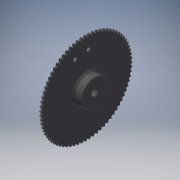
# Autodesk Inventor part: NK35B75_()
Saved by Autodesk Inventor 2018 (Build 220112000, 112)
## iProperties
Category: PARTsolutions
Company: KANA
Created: 2017-10-03
Part Number: NK35B75_()
Catalog Web Link: www.cadenas.de
Description: NK35B-Un-finished
Vendor: KANA
Document SubType Name: Modeling
Designer: psAdmin
Manufacturer: KANA
Mass: 244.907 g
Surface Area: 898.004 cm^2
Volume: 244.907 cm^3
Density: 1 g/cm^3
Material: 一般
Appearance: PSOLRGB-175-175-175
PSOL_IDENT_0: {$CADENAS_DATA\23d-libs\kana\sprockets\chain_no_35\un_finished_sprocket_steel\b_type\nk35b.prj},164
PSOL_IDENT_1: {VTYP=3D},{NB=NK35B75_()},{LINA=NK35B75},{NN=NK35B},{DATE=04.08.2017 01:43:57},{GEOMDATE=30.03.2017
PSOL_IDENT_2: 11:05:00},{VERSION=},{LINEID=490},{LINESUBID=-1},{WBVAR=SURFT}  {NB=NK35B75_()},{LINA=NK35B75},{KT=D
PSOL_IDENT_3: UMMY},{ORDERNO=NK35B75},{TYPE=NK35B},{NOT=75},{NOTX=75.000},{DP=227.46},{DO=233},{DC=222.38},{DC2=22
PSOL_IDENT_4: 2.33},{T=4.3},{DR=5.08},{MAT=None},{MATC=},{SHAPE=W : Welding type},{SHAPENB=W},{SD=16},{SURFT=},{SU
PSOL_IDENT_5: RFTNB=},{BD=68.0},{BL=25},{GD=0},{GDX=0},{S=0},{X=4},{VS=2},{SVDEL1=12},{SVDEL4=42},{SVDEL5=5},{DCX2=
PSOL_IDENT_6: 1}
NN: NK35B
NT: Un-finished
NB: NK35B75_()
NBSYN: NK35B$NOT._($SURFT.)
LINA: NK35B75
TYPE: NK35B
NOT: 75
DP: 227.46
DO: 233
DC: 222.38
DC2: 222.33
T: 4.3
SHAPE: W : Welding type
SD: 16
SURFT: No symbol : No
SUPPLIER: KANA
ARTICLENO: NK35B75_()
BOMINFO: NK35B75
CREATOR: CADENAS GmbH
Title: NK35B75
Author: Cadenas PARTsolutions
Comments: Un-finished
Autodesk Inventor part; units mm, degrees
ref_plane "YZ Plane" through (0, 0, 0) normal (1, 0, 0) x (0, 1, 0)
ref_plane "XZ Plane" through (0, 0, 0) normal (0, 1, 0) x (-1, 0, 0)
ref_plane "XY Plane" through (0, 0, 0) normal (0, 0, 1) x (1, 0, 0)
sketch "Sketch_5" plane through (0, 0, 0) normal (0, 0, 1) x (1, 0, 0)
  line L0 (25, 0) -> (0, 0)
  line L1 (0, 8.9617) -> (0.9617, 8)
  line L2 (0.9617, 8) -> (24.0383, 8)
  line L3 (24.0383, 8) -> (25, 8.9617)
  line L4 (25, 8.9617) -> (25, 33.0383)
  line L5 (25, 33.0383) -> (24.0383, 34)
  line L6 (24.0383, 34) -> (8.3, 34)
  line L7 (8.3, 34) -> (4.3, 38)
  line L8 (4.3, 38) -> (4.3, 114.8906)
  arc A0 (4.3, 114.8906) -> (3.225, 116.5) centre (-0.3844, 112.9253) ccw
  line L9 (3.225, 116.5) -> (1.075, 116.5)
  arc A1 (1.075, 116.5) -> (0, 114.8906) centre (4.6844, 112.9253) ccw
  line L10 (0, 114.8906) -> (0, 8.9617)
  constraints: 22 end point, 4 point on circle, 2 centre point
revolve "Revolution1" add sketch "Sketch_5" angle 360 about axis through (25, 0, 0) along (1, 0, 0)
sketch "Sketch_7" plane through (2.15, 0, 0) normal (1, 0, 0) x (0, 0, -1)
  circle A0 centre (0, 0) radius 155.3333
  arc A1 (-116.4803, -2.1398) -> (-116.4678, -2.7397) centre (0, 0) ccw
  line L0 (-116.4678, -2.7397) -> (-112.3345, -4.8872)
  arc A2 (-112.0613, -9.2305) -> (-112.3345, -4.8872) centre (-113.5056, -7.1412) ccw
  line L1 (-112.0613, -9.2305) -> (-115.8928, -11.8792)
  arc A3 (-115.8928, -11.8792) -> (-115.8301, -12.4759) centre (0, 0) ccw
  line L2 (-115.8301, -12.4759) -> (-111.5316, -14.27)
  arc A4 (-110.8958, -18.5752) -> (-111.5316, -14.27) centre (-112.5099, -16.614) ccw
  line L3 (-110.8958, -18.5752) -> (-114.4923, -21.5352)
  arc A5 (-114.4923, -21.5352) -> (-114.3799, -22.1245) centre (0, 0) ccw
  line L4 (-114.3799, -22.1245) -> (-109.9463, -23.5527)
  arc A6 (-108.9526, -27.7896) -> (-109.9463, -23.5527) centre (-110.7251, -25.9703) ccw
  line L5 (-108.9526, -27.7896) -> (-112.2887, -31.0401)
  arc A7 (-112.2887, -31.0401) -> (-112.1274, -31.618) centre (0, 0) ccw
  line L6 (-112.1274, -31.618) -> (-107.5899, -32.6702)
  arc A8 (-106.2451, -36.8091) -> (-107.5899, -32.6702) centre (-108.1637, -35.1445) ccw
  line L7 (-106.2451, -36.8091) -> (-109.2976, -40.3273)
  arc A9 (-109.2976, -40.3273) -> (-109.0884, -40.8897) centre (0, 0) ccw
  line L8 (-109.0884, -40.8897) -> (-104.4788, -41.5585)
  arc A10 (-102.7924, -45.5703) -> (-104.4788, -41.5585) centre (-104.8435, -44.0721) ccw
  line L9 (-102.7924, -45.5703) -> (-105.5397, -49.3317)
  arc A11 (-105.5397, -49.3317) -> (-105.2843, -49.8746) centre (0, 0) ccw
  line L10 (-105.2843, -49.8746) -> (-100.6349, -50.1553)
  arc A12 (-98.6186, -54.0119) -> (-100.6349, -50.1553) centre (-100.7879, -52.6907) ccw
  line L11 (-98.6186, -54.0119) -> (-101.0416, -57.99)
  arc A13 (-101.0416, -57.99) -> (-100.7416, -58.5096) centre (0, 0) ccw
  line L12 (-100.7416, -58.5096) -> (-96.085, -58.4003)
  arc A14 (-93.7532, -62.0747) -> (-96.085, -58.4003) centre (-96.0254, -60.9396) ccw
  line L13 (-93.7532, -62.0747) -> (-95.8348, -66.2416)
  arc A15 (-95.8348, -66.2416) -> (-95.4924, -66.7343) centre (0, 0) ccw
  line L14 (-95.4924, -66.7343) -> (-90.8612, -66.2357)
  arc A16 (-88.2301, -69.7021) -> (-90.8612, -66.2357) centre (-90.5893, -68.7611) ccw
  line L15 (-88.2301, -69.7021) -> (-89.9557, -74.0285)
  arc A17 (-89.9557, -74.0285) -> (-89.5733, -74.4908) centre (0, 0) ccw
  line L16 (-89.5733, -74.4908) -> (-85.0001, -73.6064)
  arc A18 (-82.0881, -76.8405) -> (-85.0001, -73.6064) centre (-84.5179, -76.1002) ccw
  line L17 (-82.0881, -76.8405) -> (-83.4457, -81.2962)
  arc A19 (-83.4457, -81.2962) -> (-83.0259, -81.7249) centre (0, 0) ccw
  line L18 (-83.0259, -81.7249) -> (-78.5428, -80.4609)
  arc A20 (-75.3704, -83.44) -> (-78.5428, -80.4609) centre (-77.8535, -82.9056) ccw
  line L19 (-75.3704, -83.44) -> (-76.3503, -87.9936)
  arc A21 (-76.3503, -87.9936) -> (-75.8961, -88.3857) centre (0, 0) ccw
  line L20 (-75.8961, -88.3857) -> (-71.5345, -86.751)
  arc A22 (-68.124, -89.4542) -> (-71.5345, -86.751) centre (-70.6431, -89.1295) ccw
  line L21 (-68.124, -89.4542) -> (-68.7195, -94.0738)
  arc A23 (-68.7195, -94.0738) -> (-68.234, -94.4265) centre (0, 0) ccw
  line L22 (-68.234, -94.4265) -> (-64.0245, -92.4326)
  arc A24 (-60.3997, -94.8409) -> (-64.0245, -92.4326) centre (-62.9372, -94.7281) ccw
  line L23 (-60.3997, -94.8409) -> (-60.6066, -99.4942)
  arc A25 (-60.6066, -99.4942) -> (-60.0933, -99.805) centre (0, 0) ccw
  line L24 (-60.0933, -99.805) -> (-56.0654, -97.4659)
  arc A26 (-52.2518, -99.5624) -> (-56.0654, -97.4659) centre (-54.7898, -99.6624) ccw
  line L25 (-52.2518, -99.5624) -> (-52.0685, -104.2167)
  arc A27 (-52.0685, -104.2167) -> (-51.5311, -104.4835) centre (0, 0) ccw
  line L26 (-51.5311, -104.4835) -> (-47.713, -101.8155)
  arc A28 (-43.7374, -103.5856) -> (-47.713, -101.8155) centre (-46.2582, -103.8975) ccw
  line L27 (-43.7374, -103.5856) -> (-43.1653, -108.2082)
  arc A29 (-43.1653, -108.2082) -> (-42.6074, -108.429) centre (0, 0) ccw
  line L28 (-42.6074, -108.429) -> (-39.026, -105.4509)
  arc A30 (-34.9162, -106.8821) -> (-39.026, -105.4509) centre (-37.402, -107.4039) ccw
  line L29 (-34.9162, -106.8821) -> (-33.9593, -111.4406)
  arc A31 (-33.9593, -111.4406) -> (-33.3849, -111.6141) centre (0, 0) ccw
  line L30 (-33.3849, -111.6141) -> (-30.0652, -108.3467)
  arc A32 (-25.8501, -109.429) -> (-30.0652, -108.3467) centre (-28.2835, -110.157) ccw
  line L31 (-25.8501, -109.429) -> (-24.5151, -113.8914)
  arc A33 (-24.5151, -113.8914) -> (-23.9282, -114.0162) centre (0, 0) ccw
  line L32 (-23.9282, -114.0162) -> (-20.8936, -110.4825)
  arc A34 (-16.6026, -111.2083) -> (-20.8936, -110.4825) centre (-18.9666, -112.1373) ccw
  line L33 (-16.6026, -111.2083) -> (-14.8989, -115.5434)
  arc A35 (-14.8989, -115.5434) -> (-14.3036, -115.6186) centre (0, 0) ccw
  line L34 (-14.3036, -115.6186) -> (-11.5754, -111.8434)
  arc A36 (-7.2387, -112.2075) -> (-11.5754, -111.8434) centre (-9.5167, -113.3311) ccw
  line L35 (-7.2387, -112.2075) -> (-5.1782, -116.3849)
  arc A37 (-5.1782, -116.3849) -> (-4.5788, -116.41) centre (0, 0) ccw
  line L36 (-4.5788, -116.41) -> (-2.1759, -112.4197)
  arc A38 (2.1759, -112.4197) -> (-2.1759, -112.4197) centre (0, -113.73) ccw
  line L37 (2.1759, -112.4197) -> (4.5788, -116.41)
  arc A39 (4.5788, -116.41) -> (5.1782, -116.3849) centre (0, 0) ccw
  line L38 (5.1782, -116.3849) -> (7.2387, -112.2075)
  arc A40 (11.5754, -111.8434) -> (7.2387, -112.2075) centre (9.5167, -113.3311) ccw
  line L39 (11.5754, -111.8434) -> (14.3036, -115.6186)
  arc A41 (14.3036, -115.6186) -> (14.8989, -115.5434) centre (0, 0) ccw
  line L40 (14.8989, -115.5434) -> (16.6026, -111.2083)
  arc A42 (20.8936, -110.4825) -> (16.6026, -111.2083) centre (18.9666, -112.1373) ccw
  line L41 (20.8936, -110.4825) -> (23.9282, -114.0162)
  arc A43 (23.9282, -114.0162) -> (24.5151, -113.8914) centre (0, 0) ccw
  line L42 (24.5151, -113.8914) -> (25.8501, -109.429)
  arc A44 (30.0652, -108.3467) -> (25.8501, -109.429) centre (28.2835, -110.157) ccw
  line L43 (30.0652, -108.3467) -> (33.3849, -111.6141)
  arc A45 (33.3849, -111.6141) -> (33.9593, -111.4406) centre (0, 0) ccw
  line L44 (33.9593, -111.4406) -> (34.9162, -106.8821)
  arc A46 (39.026, -105.4509) -> (34.9162, -106.8821) centre (37.402, -107.4039) ccw
  line L45 (39.026, -105.4509) -> (42.6074, -108.429)
  arc A47 (42.6074, -108.429) -> (43.1653, -108.2082) centre (0, 0) ccw
  line L46 (43.1653, -108.2082) -> (43.7374, -103.5856)
  arc A48 (47.713, -101.8155) -> (43.7374, -103.5856) centre (46.2582, -103.8975) ccw
  line L47 (47.713, -101.8155) -> (51.5311, -104.4835)
  arc A49 (51.5311, -104.4835) -> (52.0685, -104.2167) centre (0, 0) ccw
  line L48 (52.0685, -104.2167) -> (52.2518, -99.5624)
  arc A50 (56.0654, -97.4659) -> (52.2518, -99.5624) centre (54.7898, -99.6624) ccw
  line L49 (56.0654, -97.4659) -> (60.0933, -99.805)
  arc A51 (60.0933, -99.805) -> (60.6066, -99.4942) centre (0, 0) ccw
  line L50 (60.6066, -99.4942) -> (60.3997, -94.8409)
  arc A52 (64.0245, -92.4326) -> (60.3997, -94.8409) centre (62.9372, -94.7281) ccw
  line L51 (64.0245, -92.4326) -> (68.234, -94.4265)
  arc A53 (68.234, -94.4265) -> (68.7195, -94.0738) centre (0, 0) ccw
  line L52 (68.7195, -94.0738) -> (68.124, -89.4542)
  arc A54 (71.5345, -86.751) -> (68.124, -89.4542) centre (70.6431, -89.1295) ccw
  line L53 (71.5345, -86.751) -> (75.8961, -88.3857)
  arc A55 (75.8961, -88.3857) -> (76.3503, -87.9936) centre (0, 0) ccw
  line L54 (76.3503, -87.9936) -> (75.3704, -83.44)
  arc A56 (78.5428, -80.4609) -> (75.3704, -83.44) centre (77.8535, -82.9056) ccw
  line L55 (78.5428, -80.4609) -> (83.0259, -81.7249)
  arc A57 (83.0259, -81.7249) -> (83.4457, -81.2962) centre (0, 0) ccw
  line L56 (83.4457, -81.2962) -> (82.0881, -76.8405)
  arc A58 (85.0001, -73.6064) -> (82.0881, -76.8405) centre (84.5179, -76.1002) ccw
  line L57 (85.0001, -73.6064) -> (89.5733, -74.4908)
  arc A59 (89.5733, -74.4908) -> (89.9557, -74.0285) centre (0, 0) ccw
  line L58 (89.9557, -74.0285) -> (88.2301, -69.7021)
  arc A60 (90.8612, -66.2357) -> (88.2301, -69.7021) centre (90.5893, -68.7611) ccw
  line L59 (90.8612, -66.2357) -> (95.4924, -66.7343)
  arc A61 (95.4924, -66.7343) -> (95.8348, -66.2416) centre (0, 0) ccw
  line L60 (95.8348, -66.2416) -> (93.7532, -62.0747)
  arc A62 (96.085, -58.4003) -> (93.7532, -62.0747) centre (96.0254, -60.9396) ccw
  line L61 (96.085, -58.4003) -> (100.7416, -58.5096)
  arc A63 (100.7416, -58.5096) -> (101.0416, -57.99) centre (0, 0) ccw
  line L62 (101.0416, -57.99) -> (98.6186, -54.0119)
  arc A64 (100.6349, -50.1553) -> (98.6186, -54.0119) centre (100.7879, -52.6907) ccw
  line L63 (100.6349, -50.1553) -> (105.2843, -49.8746)
  arc A65 (105.2843, -49.8746) -> (105.5397, -49.3317) centre (0, 0) ccw
  line L64 (105.5397, -49.3317) -> (102.7924, -45.5703)
  arc A66 (104.4788, -41.5585) -> (102.7924, -45.5703) centre (104.8435, -44.0721) ccw
  line L65 (104.4788, -41.5585) -> (109.0884, -40.8897)
  arc A67 (109.0884, -40.8897) -> (109.2976, -40.3273) centre (0, 0) ccw
  line L66 (109.2976, -40.3273) -> (106.2451, -36.8091)
  arc A68 (107.5899, -32.6702) -> (106.2451, -36.8091) centre (108.1637, -35.1445) ccw
  line L67 (107.5899, -32.6702) -> (112.1274, -31.618)
  arc A69 (112.1274, -31.618) -> (112.2887, -31.0401) centre (0, 0) ccw
  line L68 (112.2887, -31.0401) -> (108.9526, -27.7896)
  arc A70 (109.9463, -23.5527) -> (108.9526, -27.7896) centre (110.7251, -25.9703) ccw
  line L69 (109.9463, -23.5527) -> (114.3799, -22.1245)
  arc A71 (114.3799, -22.1245) -> (114.4923, -21.5352) centre (0, 0) ccw
  line L70 (114.4923, -21.5352) -> (110.8958, -18.5752)
  arc A72 (111.5316, -14.27) -> (110.8958, -18.5752) centre (112.5099, -16.614) ccw
  line L71 (111.5316, -14.27) -> (115.8301, -12.4759)
  arc A73 (115.8301, -12.4759) -> (115.8928, -11.8792) centre (0, 0) ccw
  line L72 (115.8928, -11.8792) -> (112.0613, -9.2305)
  arc A74 (112.3345, -4.8872) -> (112.0613, -9.2305) centre (113.5056, -7.1412) ccw
  line L73 (112.3345, -4.8872) -> (116.4678, -2.7397)
  arc A75 (116.4678, -2.7397) -> (116.4803, -2.1398) centre (0, 0) ccw
  line L74 (116.4803, -2.1398) -> (112.4406, 0.1789)
  arc A76 (112.3495, 4.5298) -> (112.4406, 0.1789) centre (113.7051, 2.3818) ccw
  line L75 (112.3495, 4.5298) -> (116.2886, 7.0157)
  arc A77 (116.2886, 7.0157) -> (116.2509, 7.6145) centre (0, 0) ccw
  line L76 (116.2509, 7.6145) -> (112.0313, 9.587)
  arc A78 (111.5764, 13.9151) -> (112.0313, 9.587) centre (113.107, 11.888) ccw
  line L77 (111.5764, 13.9151) -> (115.2937, 16.7218)
  arc A79 (115.2937, 16.7218) -> (115.206, 17.3154) centre (0, 0) ccw
  line L78 (115.206, 17.3154) -> (110.8362, 18.9279)
  arc A80 (110.0207, 23.2028) -> (110.8362, 18.9279) centre (111.7155, 21.3109) ccw
  line L79 (110.0207, 23.2028) -> (113.4901, 26.3107)
  arc A81 (113.4901, 26.3107) -> (113.3531, 26.8949) centre (0, 0) ccw
  line L80 (113.3531, 26.8949) -> (108.8636, 28.1361)
  arc A82 (107.6933, 32.3277) -> (108.8636, 28.1361) centre (109.5405, 30.5843) ccw
  line L81 (107.6933, 32.3277) -> (110.8904, 35.715)
  arc A83 (110.8904, 35.715) -> (110.705, 36.2857) centre (0, 0) ccw
  line L82 (110.705, 36.2857) -> (106.1274, 37.1469)
  arc A84 (104.6105, 41.2258) -> (106.1274, 37.1469) centre (106.5971, 39.6431) ccw
  line L83 (104.6105, 41.2258) -> (107.513, 44.8689)
  arc A85 (107.513, 44.8689) -> (107.2804, 45.422) centre (0, 0) ccw
  line L84 (107.2804, 45.422) -> (102.6469, 45.8971)
  arc A86 (100.7939, 49.8348) -> (102.6469, 45.8971) centre (102.906, 48.4239) ccw
  line L85 (100.7939, 49.8348) -> (103.3814, 53.7079)
  arc A87 (103.3814, 53.7079) -> (103.1034, 54.2397) centre (0, 0) ccw
  line L86 (103.1034, 54.2397) -> (98.4463, 54.3254)
  arc A88 (96.2704, 58.0943) -> (98.4463, 54.3254) centre (98.4931, 56.865) ccw
  line L87 (96.2704, 58.0943) -> (98.5246, 62.1703)
  arc A89 (98.5246, 62.1703) -> (98.2031, 62.6769) centre (0, 0) ccw
  line L88 (98.2031, 62.6769) -> (93.5552, 62.3727)
  arc A90 (91.0715, 65.9462) -> (93.5552, 62.3727) centre (93.3893, 64.9073) ccw
  line L89 (91.0715, 65.9462) -> (92.9768, 70.1966)
  arc A91 (92.9768, 70.1966) -> (92.614, 70.6745) centre (0, 0) ccw
  line L90 (92.614, 70.6745) -> (88.0079, 69.9824)
  arc A92 (85.2339, 73.3356) -> (88.0079, 69.9824) centre (87.6305, 72.4942) ccw
  line L91 (85.2339, 73.3356) -> (86.7768, 77.7305)
  arc A93 (86.7768, 77.7305) -> (86.3753, 78.1764) centre (0, 0) ccw
  line L92 (86.3753, 78.1764) -> (81.8432, 77.1013)
  arc A94 (78.7984, 80.2106) -> (81.8432, 77.1013) centre (81.257, 79.5727) ccw
  line L93 (78.7984, 80.2106) -> (79.9682, 84.7192)
  arc A95 (79.9682, 84.7192) -> (79.5308, 85.1299) centre (0, 0) ccw
  line L94 (79.5308, 85.1299) -> (75.1045, 83.6794)
  arc A96 (71.8102, 86.523) -> (75.1045, 83.6794) centre (74.3135, 86.093) ccw
  line L95 (71.8102, 86.523) -> (72.5986, 91.1136)
  arc A97 (72.5986, 91.1136) -> (72.1284, 91.4863) centre (0, 0) ccw
  line L96 (72.1284, 91.4863) -> (67.839, 89.6705)
  arc A98 (64.3183, 92.2284) -> (67.839, 89.6705) centre (66.8488, 92.0095) ccw
  line L97 (64.3183, 92.2284) -> (64.7198, 96.869)
  arc A99 (64.7198, 96.869) -> (64.22, 97.201) centre (0, 0) ccw
  line L98 (64.22, 97.201) -> (60.0977, 95.0326)
  arc A100 (56.3752, 97.287) -> (60.0977, 95.0326) centre (58.9152, 97.2806) ccw
  line L99 (56.3752, 97.287) -> (56.387, 101.9449)
  arc A101 (56.387, 101.9449) -> (55.8612, 102.2339) centre (0, 0) ccw
  line L100 (55.8612, 102.2339) -> (51.9348, 99.7282)
  arc A102 (48.0367, 101.6632) -> (51.9348, 99.7282) centre (50.5684, 101.8693) ccw
  line L101 (48.0367, 101.6632) -> (47.6587, 106.3057)
  arc A103 (47.6587, 106.3057) -> (47.1106, 106.5497) centre (0, 0) ccw
  line L102 (47.1106, 106.5497) -> (43.4076, 103.7242)
  arc A104 (39.3613, 105.3262) -> (43.4076, 103.7242) centre (41.8668, 105.7435) ccw
  line L103 (39.3613, 105.3262) -> (38.5962, 109.9208)
  arc A105 (38.5962, 109.9208) -> (38.0295, 110.1181) centre (0, 0) ccw
  line L104 (38.0295, 110.1181) -> (34.576, 106.9927)
  arc A106 (30.4098, 108.2505) -> (34.576, 106.9927) centre (32.8716, 108.8759) ccw
  line L105 (30.4098, 108.2505) -> (29.2629, 112.765)
  arc A107 (29.2629, 112.765) -> (28.6817, 112.9142) centre (0, 0) ccw
  line L106 (28.6817, 112.9142) -> (25.5018, 109.5107)
  arc A108 (21.245, 110.4155) -> (25.5018, 109.5107) centre (23.6458, 111.2447) ccw
  line L107 (21.245, 110.4155) -> (19.7243, 114.8181)
  arc A109 (19.7243, 114.8181) -> (19.1327, 114.9182) centre (0, 0) ccw
  line L108 (19.1327, 114.9182) -> (16.2487, 111.2605)
  arc A110 (11.9311, 111.806) -> (16.2487, 111.2605) centre (14.2541, 112.8332) ccw
  line L109 (11.9311, 111.806) -> (10.0474, 116.0659)
  arc A111 (10.0474, 116.0659) -> (9.4495, 116.1161) centre (0, 0) ccw
  line L110 (9.4495, 116.1161) -> (6.8817, 112.23)
  arc A112 (2.5336, 112.4122) -> (6.8817, 112.23) centre (4.7625, 113.6302) ccw
  line L111 (2.5336, 112.4122) -> (0.3, 116.4996)
  arc A113 (0.3, 116.4996) -> (-0.3, 116.4996) centre (0, 0) ccw
  line L112 (-0.3, 116.4996) -> (-2.5336, 112.4122)
  arc A114 (-6.8817, 112.23) -> (-2.5336, 112.4122) centre (-4.7625, 113.6302) ccw
  line L113 (-6.8817, 112.23) -> (-9.4495, 116.1161)
  arc A115 (-9.4495, 116.1161) -> (-10.0474, 116.0659) centre (0, 0) ccw
  line L114 (-10.0474, 116.0659) -> (-11.9311, 111.806)
  arc A116 (-16.2487, 111.2605) -> (-11.9311, 111.806) centre (-14.2541, 112.8332) ccw
  line L115 (-16.2487, 111.2605) -> (-19.1327, 114.9182)
  arc A117 (-19.1327, 114.9182) -> (-19.7243, 114.8181) centre (0, 0) ccw
  line L116 (-19.7243, 114.8181) -> (-21.245, 110.4155)
  arc A118 (-25.5018, 109.5107) -> (-21.245, 110.4155) centre (-23.6458, 111.2447) ccw
  line L117 (-25.5018, 109.5107) -> (-28.6817, 112.9142)
  arc A119 (-28.6817, 112.9142) -> (-29.2629, 112.765) centre (0, 0) ccw
  line L118 (-29.2629, 112.765) -> (-30.4098, 108.2505)
  arc A120 (-34.576, 106.9927) -> (-30.4098, 108.2505) centre (-32.8716, 108.8759) ccw
  line L119 (-34.576, 106.9927) -> (-38.0295, 110.1181)
  arc A121 (-38.0295, 110.1181) -> (-38.5962, 109.9208) centre (0, 0) ccw
  line L120 (-38.5962, 109.9208) -> (-39.3613, 105.3262)
  arc A122 (-43.4076, 103.7242) -> (-39.3613, 105.3262) centre (-41.8668, 105.7435) ccw
  line L121 (-43.4076, 103.7242) -> (-47.1106, 106.5497)
  arc A123 (-47.1106, 106.5497) -> (-47.6587, 106.3057) centre (0, 0) ccw
  line L122 (-47.6587, 106.3057) -> (-48.0367, 101.6632)
  arc A124 (-51.9348, 99.7282) -> (-48.0367, 101.6632) centre (-50.5684, 101.8693) ccw
  line L123 (-51.9348, 99.7282) -> (-55.8612, 102.2339)
  arc A125 (-55.8612, 102.2339) -> (-56.387, 101.9449) centre (0, 0) ccw
  line L124 (-56.387, 101.9449) -> (-56.3752, 97.287)
  arc A126 (-60.0977, 95.0326) -> (-56.3752, 97.287) centre (-58.9152, 97.2806) ccw
  line L125 (-60.0977, 95.0326) -> (-64.22, 97.201)
  arc A127 (-64.22, 97.201) -> (-64.7198, 96.869) centre (0, 0) ccw
  line L126 (-64.7198, 96.869) -> (-64.3183, 92.2284)
  arc A128 (-67.839, 89.6705) -> (-64.3183, 92.2284) centre (-66.8488, 92.0095) ccw
  line L127 (-67.839, 89.6705) -> (-72.1284, 91.4863)
  arc A129 (-72.1284, 91.4863) -> (-72.5986, 91.1136) centre (0, 0) ccw
  line L128 (-72.5986, 91.1136) -> (-71.8102, 86.523)
  arc A130 (-75.1045, 83.6794) -> (-71.8102, 86.523) centre (-74.3135, 86.093) ccw
  line L129 (-75.1045, 83.6794) -> (-79.5308, 85.1299)
  arc A131 (-79.5308, 85.1299) -> (-79.9682, 84.7192) centre (0, 0) ccw
  line L130 (-79.9682, 84.7192) -> (-78.7984, 80.2106)
  arc A132 (-81.8432, 77.1013) -> (-78.7984, 80.2106) centre (-81.257, 79.5727) ccw
  line L131 (-81.8432, 77.1013) -> (-86.3753, 78.1764)
  arc A133 (-86.3753, 78.1764) -> (-86.7768, 77.7305) centre (0, 0) ccw
  line L132 (-86.7768, 77.7305) -> (-85.2339, 73.3356)
  arc A134 (-88.0079, 69.9824) -> (-85.2339, 73.3356) centre (-87.6305, 72.4942) ccw
  line L133 (-88.0079, 69.9824) -> (-92.614, 70.6745)
  arc A135 (-92.614, 70.6745) -> (-92.9768, 70.1966) centre (0, 0) ccw
  line L134 (-92.9768, 70.1966) -> (-91.0715, 65.9462)
  arc A136 (-93.5552, 62.3727) -> (-91.0715, 65.9462) centre (-93.3893, 64.9073) ccw
  line L135 (-93.5552, 62.3727) -> (-98.2031, 62.6769)
  arc A137 (-98.2031, 62.6769) -> (-98.5246, 62.1703) centre (0, 0) ccw
  line L136 (-98.5246, 62.1703) -> (-96.2704, 58.0943)
  arc A138 (-98.4463, 54.3254) -> (-96.2704, 58.0943) centre (-98.4931, 56.865) ccw
  line L137 (-98.4463, 54.3254) -> (-103.1034, 54.2397)
  arc A139 (-103.1034, 54.2397) -> (-103.3814, 53.7079) centre (0, 0) ccw
  line L138 (-103.3814, 53.7079) -> (-100.7939, 49.8348)
  arc A140 (-102.6469, 45.8971) -> (-100.7939, 49.8348) centre (-102.906, 48.4239) ccw
  line L139 (-102.6469, 45.8971) -> (-107.2804, 45.422)
  arc A141 (-107.2804, 45.422) -> (-107.513, 44.8689) centre (0, 0) ccw
  line L140 (-107.513, 44.8689) -> (-104.6105, 41.2258)
  arc A142 (-106.1274, 37.1469) -> (-104.6105, 41.2258) centre (-106.5971, 39.6431) ccw
  line L141 (-106.1274, 37.1469) -> (-110.705, 36.2857)
  arc A143 (-110.705, 36.2857) -> (-110.8904, 35.715) centre (0, 0) ccw
  line L142 (-110.8904, 35.715) -> (-107.6933, 32.3277)
  arc A144 (-108.8636, 28.1361) -> (-107.6933, 32.3277) centre (-109.5405, 30.5843) ccw
  line L143 (-108.8636, 28.1361) -> (-113.3531, 26.8949)
  arc A145 (-113.3531, 26.8949) -> (-113.4901, 26.3107) centre (0, 0) ccw
  line L144 (-113.4901, 26.3107) -> (-110.0207, 23.2028)
  arc A146 (-110.8362, 18.9279) -> (-110.0207, 23.2028) centre (-111.7155, 21.3109) ccw
  line L145 (-110.8362, 18.9279) -> (-115.206, 17.3154)
  arc A147 (-115.206, 17.3154) -> (-115.2937, 16.7218) centre (0, 0) ccw
  line L146 (-115.2937, 16.7218) -> (-111.5764, 13.9151)
  arc A148 (-112.0313, 9.587) -> (-111.5764, 13.9151) centre (-113.107, 11.888) ccw
  line L147 (-112.0313, 9.587) -> (-116.2509, 7.6145)
  arc A149 (-116.2509, 7.6145) -> (-116.2886, 7.0157) centre (0, 0) ccw
  line L148 (-116.2886, 7.0157) -> (-112.3495, 4.5298)
  arc A150 (-112.4406, 0.1789) -> (-112.3495, 4.5298) centre (-113.7051, 2.3818) ccw
  line L149 (-112.4406, 0.1789) -> (-116.4803, -2.1398)
  constraints: 300 end point, 300 point on circle, 151 centre point
extrude "Extrusion1" cut sketch "Sketch_7" along normal mid plane 4.7
ref_plane "body_XY" through (0, 0, 0) normal (1, 0, 0) x (0, 0, -1)
ref_plane "body_YZ" through (0, 0, 0) normal (0, 0, -1) x (0, 1, 0)
ref_plane "body_ZX" through (0, 0, 0) normal (0, 1, 0) x (1, 0, 0)
sketch "スケッチ3" plane through (4.3, 0, 0) normal (1, 0, 0) x (0, 0.146083, -0.9892723)
  circle A0 centre (0, 0) radius 82
  circle A1 centre (0, 0) radius 80.206
  line L0 (-80.206, -17.0587) -> (-80.206, 17.0587)
  line L1 (-80.206, 0) -> (-46.2537, 0) construction
  dimension "d5" = 160.412
  dimension "d4" = 164
  dimension "d6" = 90
  constraints: 4 coincident, 4 end point, 2 point on circle, 1 centre point, 1 horizontal, 1 horizontal alignment, 1 midpoint, 2 other
  measures "d4" diameter of A0
  measures "d6" angle of L1 L0
hole "穴1" at (4.3, 5.1589, 81.8376) at (4.3, -28.5924, 76.8536) direction (-1, 0, 0) diameter 10 end through all
body "Solid1"
